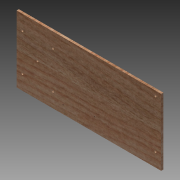
# Autodesk Inventor part: bed support
Saved by Autodesk Inventor 2015 (Build 190159000, 159)
## iProperties
Created: 2015-07-09
Part Number: bed support
Material: Wood (Birch)
Document SubType Name: Modeling
Designer: hp
Density: 0.55 g/cm^3
Appearance: Birch - Natural Polished
Author: hp
Autodesk Inventor part; units mm, degrees
ref_plane "YZ Plane" through (0, 0, 0) normal (1, 0, 0) x (0, 1, 0)
ref_plane "XZ Plane" through (0, 0, 0) normal (0, 1, 0) x (-1, 0, 0)
ref_plane "XY Plane" through (0, 0, 0) normal (0, 0, 1) x (1, 0, 0)
sketch "Sketch1" plane through (0, 0, 0) normal (0, 1, 0) x (-1, 0, 0)
  line L0 (0, 60) -> (-260, 60)
  line L1 (-260, 60) -> (-260, -60)
  line L2 (-260, -60) -> (0, -60)
  line L3 (0, -60) -> (0, 60)
  circle A0 centre (-10, 33.5) radius 2
  circle A1 centre (-10, -33.5) radius 2
  circle A2 centre (-65, 33.5) radius 2
  circle A3 centre (-65, -33.5) radius 2
  circle A4 centre (-37.05, 0) radius 2
  circle A5 centre (-249.5, 51.6) radius 2
  circle A6 centre (-249.5, -35.26) radius 2
  point P0 (0, 0)
  point P1 (0, 0)
  dimension "d2" = 260
  dimension "d3" = 120
  dimension "d4" = 4
  dimension "d5" = 55
  dimension "d6" = 67
  dimension "d7" = 33.5
  dimension "d8" = 10
  dimension "d11" = 4
  dimension "d13" = 37.05
  dimension "d14" = 4
  dimension "d15" = 4
  dimension "d17" = 10.5
  dimension "d18" = 24.74
  dimension "d19" = 8.4
  constraints: 8 end point, 7 centre point, 4 vertical alignment, 3 equal radius, 3 horizontal alignment, 2 parallel, 1 coincident, 1 horizontal, 1 midpoint, 1 perpendicular
  measures "d2" distance of L2.end L1.end
  measures "d3" distance of L1.end L0.end
  measures "d4" diameter of A0
  measures "d5" distance of A2.centre A0.centre
  measures "d6" distance of A1.centre A0.centre
  measures "d7" vertical distance of point (0, 0) A0.centre
  measures "d8" distance from line of L3 A0.centre
  measures "d11" diameter of A4
  measures "d13" distance of point (0, 0) A4.centre
  measures "d14" diameter of A5
  measures "d15" diameter of A6
  measures "d17" distance from line of A5.centre L1
  measures "d18" distance from line of L2 A6.centre
  measures "d19" distance from line of A5.centre L0
extrude "Extrusion2" add sketch "Sketch1" along normal blind 4
equation "\"d7\" = 0.5 * d6"
body "Solid2"
